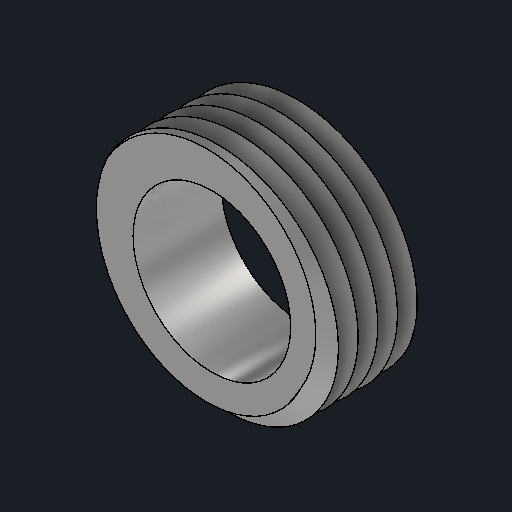
# Autodesk Inventor part: Rod
Saved by Autodesk Inventor 2026.2 (Build 302298000, 298)
## iProperties
Created: 2015-04-29
Part Number: Rod
Material: Stainless Steel
Document SubType Name: Modeling
Designer: Philip
Density: 8 g/cm^3
Appearance: Semi-Polished
Author: Philip
Autodesk Inventor part; units mm, degrees
ref_plane "YZ Plane" through (0, 0, 0) normal (1, 0, 0) x (0, 1, 0)
ref_plane "XZ Plane" through (0, 0, 0) normal (0, 1, 0) x (-1, 0, 0)
ref_plane "XY Plane" through (0, 0, 0) normal (0, 0, 1) x (1, 0, 0)
sketch "Sketch1" plane through (0, 0, 0) normal (0, 0, 1) x (1, 0, 0)
  circle A0 centre (0, 0) radius 4.7625
  dimension "d0" = 9.525
  constraints: 1 centre point, 1 coincident
  measures "d0" diameter of A0
extrude "Extrusion1" add sketch "Sketch1" along normal blind 3.556
sketch "Sketch2" plane through (0, 0, 0) normal (0, 1, 0) x (-1, 0, 0)
  line L0 (4.7625, 4.4126) -> (4.0751, 4.0157)
  line L1 (4.0751, 4.0157) -> (4.7625, 3.6189)
  line L2 (4.7625, 3.6189) -> (4.7625, 4.4126)
  line L3 (4.7625, 0) -> (4.7625, 3.556) projected
  point P0 (0, 0)
  dimension "d3" = 60
  dimension "d4" = 0.7937
  dimension "d5" = 0.3969
  constraints: 6 end point, 1 collinear
  measures "d3" angle of L1 L0
  measures "d4" distance of L0.start L1.end
  measures "d5" vertical distance of L1.end L0.end
coil "Coil1" sketch "Sketch2" operation cut axis through (0, 0, -10) along (0, 0, -1) pitch 0.7937 turns 7 hand right
sketch "Sketch3" plane through (0, 0, 3.556) normal (0, 0, 1) x (1, 0, 0)
  point P0 (0, 0)
  point P1 (0, 0)
  constraints: 1 coincident
hole "Hole1" at (0, 0, 3.556) direction (0, 0, -1) diameter 6.35 end through all
equation "\"d5\" = 0.5 * d4"
body "Solid1"
